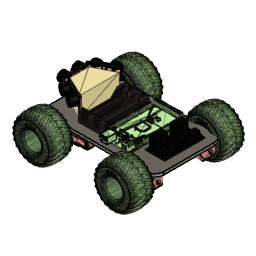
ROBOCAR v0 (Autodesk Fusion 360 design; units mm, degrees)
Autodesk Fusion 360 part; units mm, degrees
sketch "Sketch1" plane through (0, 0, 0) normal (0, 0, 1) x (1, 0, 0)
  line L0 (15, 0) -> (182.6791, 0)
  line L1 (197.6791, 15) -> (197.6791, 101.6916)
  line L2 (182.6791, 116.6916) -> (15, 116.6916)
  line L3 (0, 101.6916) -> (0, 15)
  arc A0 (0, 15) -> (15, 0) centre (15, 15) ccw
  arc A1 (15, 116.6916) -> (0, 101.6916) centre (15, 101.6916) ccw
  arc A2 (197.6791, 101.6916) -> (182.6791, 116.6916) centre (182.6791, 101.6916) ccw
  arc A3 (182.6791, 0) -> (197.6791, 15) centre (182.6791, 15) ccw
  dimension "d1" = 15
  dimension "d2" = 15
  dimension "d3" = 15
  dimension "d4" = 15
  constraint horizontal L0
  constraint vertical L1
  constraint horizontal L2
  constraint vertical L3
  constraint tangent L0 A0
  constraint tangent L3 A0
  constraint tangent L2 A1
  constraint tangent L3 A1
  constraint tangent L1 A2
  constraint tangent L2 A2
  constraint tangent L0 A3
  constraint tangent L1 A3
  measures "d1" radius of A0
  measures "d2" radius of A1
  measures "d3" radius of A2
  measures "d4" radius of A3
extrude "Extrude1" add sketch "Sketch1" along normal blind 5
other "Base Mesh Feature1"
other "CopyPasteMeshes1"
other "Modify1"
other "Modify2"
other "Modify3"
other "Modify4"
other "Modify5"
other "Modify6"
other "Modify7"
other "CopyPasteMeshes2"
other "Modify8"
other "CopyPasteMeshes3"
other "Modify9"
other "Base Mesh Feature2"
other "Modify10"
other "Modify11"
other "CopyPasteMeshes4"
other "Modify12"
other "Modify13"
other "CopyPasteMeshes5"
other "Modify14"
other "Modify15"
other "Modify16"
other "Modify17"
other "Modify18"
other "Modify19"
other "Modify20"
other "Base Mesh Feature4"
other "Scale1"
other "Modify24"
other "Modify25"
other "MeshRepair1"
other "Modify26"
other "Modify27"
other "CopyPasteMeshes6"
other "Modify28"
other "Modify29"
other "Modify30"
other "Modify31"
other "Base Mesh Feature5"
other "Modify34"
other "Modify35"
other "Modify36"
other "Modify37"
other "Modify38"
other "Modify39"
other "Modify40"
other "Modify41"
other "Modify42"
other "Base Mesh Feature6"
other "Modify43"
other "Modify44"
other "CopyPasteMeshes7"
other "Modify45"
other "CopyPasteMeshes8"
other "Modify46"
other "CopyPasteMeshes9"
other "Modify47"
other "Modify48"
other "Modify49"
other "Modify50"
other "Modify51"
other "Modify52"
sketch "Sketch2" plane through (0, 0, 0) normal (0, 0, 1) x (1, 0, 0)
other "MeshRepair3"
other "Modify54"
other "Modify56"
other "Base Mesh Feature8"
other "Scale2"
other "Modify60"
other "Modify61"
other "Modify62"
other "Modify63"
other "Modify64"
other "Modify65"
other "Modify66"
other "Modify67"
other "Modify68"
other "Modify69"
other "Modify70"
other "Modify71"
other "Modify72"
other "Modify73"
other "Modify74"
other "Modify75"
other "Modify76"
other "Modify77"
other "Base Mesh Feature9"
other "Modify78"
other "Modify79"
other "Modify80"
other "Modify81"
other "Modify82"
other "Modify83"
other "Modify84"
other "Modify85"
other "Modify86"
other "CopyPasteMeshes10"
